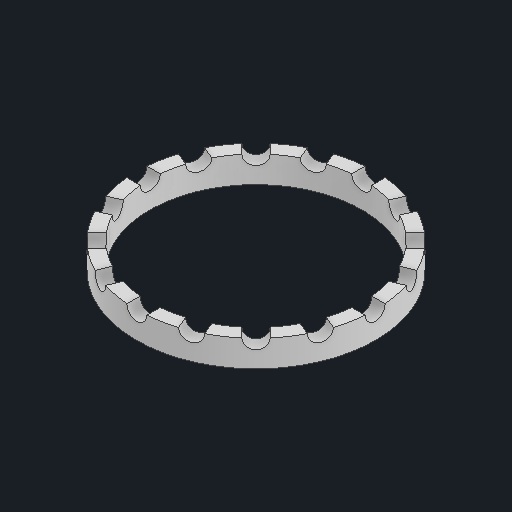
# Autodesk Inventor part: CastleSpacer
Saved by Autodesk Inventor 2024 (Build 280153000, 153)
## iProperties
Created: 2025-02-07
Part Number: CastleSpacer
Material: Generic
Document SubType Name: Modeling
Designer: Tommy Rohmann
Density: 1 g/cm^3
Appearance: Default
Author: Tommy Rohmann
Autodesk Inventor part; units mm, degrees
ref_plane "YZ Plane" through (0, 0, 0) normal (1, 0, 0) x (0, 1, 0)
ref_plane "XZ Plane" through (0, 0, 0) normal (0, 1, 0) x (-1, 0, 0)
ref_plane "XY Plane" through (0, 0, 0) normal (0, 0, 1) x (1, 0, 0)
sketch "CastleSpacer" plane through (0, 0, 0) normal (0, 0, 1) x (1, 0, 0)
  line L0 (50.8, -9.4801) -> (50.8, -9.4801)
  line L1 (50.8, -9.4801) -> (57.15, -9.4801)
  line L2 (57.15, -9.4801) -> (57.15, -9.4801)
  line L3 (57.15, -9.4801) -> (50.8, -9.4801)
  line L4 (50.8, -9.4801) -> (50.8, 3.2199)
  line L5 (50.8, 3.2199) -> (57.15, 3.2199)
  line L6 (57.15, 3.2199) -> (57.15, -9.4801)
  point P0 (50.8, 0)
  dimension "d158" = 0
  dimension "d159" = 6.35
  dimension "d383" = 12.7
  measures "d158" distance of L1.end L2.end
  measures "d159" distance of L0.end L1.end
  measures "d383" distance of L0.end L4.end
derived "LAYOUT.ipt"
sketch "Sketch1" plane through (0, 0, 0) normal (0, 0, 1) x (1, 0, 0)
  line L0 (0.0116, -18.9925) -> (0.0116, 19.3875)
  line L1 (50.8116, -9.4801) -> (50.8116, -9.4801)
  line L2 (50.8116, -9.4801) -> (57.1616, -9.4801)
  line L3 (57.1616, -9.4801) -> (57.1616, -9.4801)
  line L4 (57.1616, -9.4801) -> (50.8116, -9.4801)
  line L5 (50.8116, -9.4801) -> (50.8116, 3.2199)
  line L6 (50.8116, 3.2199) -> (57.1616, 3.2199)
  line L7 (57.1616, 3.2199) -> (57.1616, -9.4801)
  point P0 (57.1616, -9.4801)
  dimension "d1" = 101.6
  constraints: 2 end point, 1 vertical
revolve "Revolution1" add sketch "Sketch1" angle 22.5 mid plane about axis through (0.0116, -18.9925, 0) along (0, 1, 0)
sketch "Sketch2" plane through (0.0116, 3.2199, 0) normal (0, 1, 0) x (1, 0, 0)
  arc A0 (56.0519, -11.1494) -> (56.0519, 11.1494) centre (0, 0) ccw projected
  line L0 (77.3841, 0) -> (32.2872, 0)
  line L1 (32.2872, 0) -> (32.2872, 4.7625)
  line L2 (32.2872, 4.7625) -> (77.3841, 4.7625)
  line L3 (77.3841, 0) -> (77.3841, 4.7625)
  point P0 (-0.0116, 0)
  point P1 (57.15, 0)
  point P2 (56.9512, 4.7625)
  dimension "d3" = 4.7625
  constraints: 8 end point, 2 perpendicular, 1 horizontal, 1 point on circle, 1 point on line, 1 vertical
  measures "d3" distance of L0.end L1.end
revolve "Revolution2" cut sketch "Sketch2" angle 360 about axis through (77.3957, 3.2199, 0) along (1, 0, 0)
pattern_circular "Circular Pattern1" count 16 over 360 about axis through (0.0116, -3.1301, 0) along (0, 1, 0)
body "Solid1"
